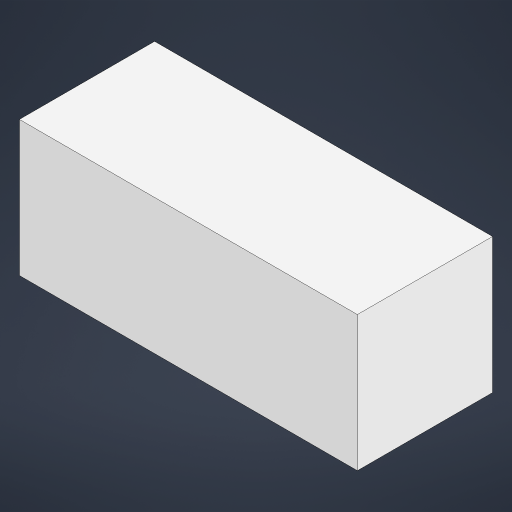
# Autodesk Inventor part: edgert
Saved by Autodesk Inventor 2023.1 (Build 271208000, 208)
## iProperties
RuleStatus: InUse
Created: 2022-09-14
Part Number: edgert
Material: Granite, Cut, Polished
Document SubType Name: Modeling
Designer: awelt
Mass: 7079.21 g
Surface Area: 1238.71 cm^2
Volume: 2621.93 cm^3
Density: 2.7 g/cm^3
Appearance: Amber Select
AfterDocSave0: Convert in3 volume to ft3
in3 to ft3: 0.09
TEST: 0.0
BoundingBL1: 4
BoundingBL2: 4
BoundingBL3: 10
BoundingCF: 0.093
Author: awelt
Autodesk Inventor part; units mm, degrees
ref_plane "YZ Plane" through (0, 0, 0) normal (1, 0, 0) x (0, 1, 0)
ref_plane "XZ Plane" through (0, 0, 0) normal (0, 1, 0) x (-1, 0, 0)
ref_plane "XY Plane" through (0, 0, 0) normal (0, 0, 1) x (1, 0, 0)
sketch "Sketch1" plane through (0, 0, 0) normal (0, 1, 0) x (-1, 0, 0)
  line L0 (0, 0) -> (-254, 0)
  line L1 (-254, 0) -> (-254, 101.6)
  line L2 (-254, 101.6) -> (0, 101.6)
  line L3 (0, 101.6) -> (0, 0)
  dimension "d0" = 254
  dimension "d1" = 101.6
  constraints: 8 end point, 2 parallel, 1 horizontal, 1 perpendicular
  measures "d0" distance of L1.end L2.end
  measures "d1" distance of L0.end L1.end
extrude "Extrusion1" add sketch "Sketch1" along normal blind 101.6
body "Solid1"
